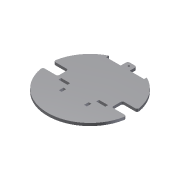
# Autodesk Inventor part: OpenROV_Dev_EChassis_Pivot_Plate
Saved by Autodesk Inventor 2012 (Build 160160000, 160)
## iProperties
Created: 2012-08-08
Part Number: OpenROV_Dev_EChassis_Pivot_Plate
Material: Default
Document SubType Name: Modeling
Designer: user
Density: 1 g/cm^3
Author: user
Autodesk Inventor part; units mm, degrees
ref_plane "YZ Plane" through (0, 0, 0) normal (1, 0, 0) x (0, 1, 0)
ref_plane "XZ Plane" through (0, 0, 0) normal (0, 1, 0) x (-1, 0, 0)
ref_plane "XY Plane" through (0, 0, 0) normal (0, 0, 1) x (1, 0, 0)
sketch "Sketch1" plane through (0, 0, 0) normal (0, 0, 1) x (1, 0, 0)
  line L0 (-26, -6) -> (-16, -6)
  line L1 (-16, -6) -> (-16, -9)
  line L2 (-16, -9) -> (-26, -9)
  line L3 (-26, -9) -> (-26, -6)
  line L4 (16, -6) -> (26, -6)
  line L5 (26, -6) -> (26, -9)
  line L6 (26, -9) -> (16, -9)
  line L7 (16, -9) -> (16, -6)
  line L8 (-15.5, -14) -> (-12.5, -14)
  line L9 (-12.5, -14) -> (-12.5, -19)
  line L10 (-12.5, -19) -> (-15.5, -19)
  line L11 (-15.5, -19) -> (-15.5, -14)
  line L12 (12.5, -14) -> (15.5, -14)
  line L13 (15.5, -14) -> (15.5, -19)
  line L14 (15.5, -19) -> (12.5, -19)
  line L15 (12.5, -19) -> (12.5, -14)
  arc A0 (31.6739, 34.7241) -> (21, 42.0476) centre (0, 0) ccw
  arc A1 (-28.2, 37.6) -> (-31.6739, 34.7241) centre (0, 0) ccw
  line L16 (21, 42.0476) -> (21, 39.0476)
  line L17 (21, 39.0476) -> (5, 39.0476)
  line L18 (-21, 42.0476) -> (-21, 39.0476)
  line L19 (-21, 39.0476) -> (-5, 39.0476)
  line L20 (-5, 39.0476) -> (-5, 44.8999)
  line L21 (5, 39.0476) -> (5, 44.8999)
  arc A2 (3.1333, 46.8954) -> (-3.1333, 46.8954) centre (0, 0) ccw
  circle A3 centre (0, 43.0476) radius 1
  arc A4 (-3.1333, 46.8954) -> (-5, 44.8999) centre (-3, 44.8999) ccw
  arc A5 (5, 44.8999) -> (3.1333, 46.8954) centre (3, 44.8999) ccw
  line L22 (-44.2832, -6) -> (-32, -6)
  line L23 (-30, -4) -> (-30, 4)
  line L24 (-32, 6) -> (-44.2832, 6)
  arc A6 (-21, 42.0476) -> (-46.2513, 8.3556) centre (0, 0) ccw
  line L25 (44.2832, 6) -> (32, 6)
  line L26 (30, 4) -> (30, -4)
  line L27 (32, -6) -> (44.2832, -6)
  arc A7 (-46.2513, -8.3556) -> (46.2513, -8.3556) centre (0, 0) ccw
  arc A8 (46.2513, 8.3556) -> (28.2, 37.6) centre (0, 0) ccw
  arc A9 (44.2832, 6) -> (46.2513, 8.3556) centre (44.2832, 8) ccw
  arc A10 (32, 6) -> (30, 4) centre (32, 4) ccw
  arc A11 (30, -4) -> (32, -6) centre (32, -4) ccw
  arc A12 (46.2513, -8.3556) -> (44.2832, -6) centre (44.2832, -8) ccw
  arc A13 (-46.2513, 8.3556) -> (-44.2832, 6) centre (-44.2832, 8) ccw
  arc A14 (-30, 4) -> (-32, 6) centre (-32, 4) ccw
  arc A15 (-32, -6) -> (-30, -4) centre (-32, -4) ccw
  arc A16 (-44.2832, -6) -> (-46.2513, -8.3556) centre (-44.2832, -8) ccw
  point P0 (-5, 46.7333)
  point P1 (5, 46.7333)
  point P2 (-46.6154, -6)
  point P3 (-46.6154, 6)
  point P4 (46.6154, -6)
  point P5 (46.6154, 6)
  dimension "d3" = 10
  dimension "d4" = 10
  dimension "d5" = 3
  dimension "d6" = 3
  dimension "d7" = 32
  dimension "d8" = 16
  dimension "d12" = 6
  dimension "d13" = 6
  dimension "d14" = 3
  dimension "d15" = 5
  dimension "d16" = 5
  dimension "d17" = 3
  dimension "d18" = 25
  dimension "d19" = 12.5
  dimension "d20" = 5
  dimension "d21" = 5
  dimension "d30" = 3
  dimension "d31" = 3
  dimension "d37" = 47
  dimension "d38" = 10
  dimension "d39" = 16
  dimension "d40" = 16
  dimension "d41" = 2
  dimension "d42" = 4
  dimension "d43" = 5
  dimension "d44" = 5
  dimension "d45" = 2
  dimension "d46" = 30
  dimension "d47" = 30
  dimension "d48" = 2
  constraints: 56 end point, 40 point on circle, 20 tangent, 17 centre point, 12 parallel, 10 perpendicular, 8 equal radius, 6 horizontal, 6 point on line, 2 coincident
  measures "d3" distance between parallel lines of L1 L3
  measures "d4" distance between parallel lines of L5 L7
  measures "d5" distance between parallel lines of L2 L0
  measures "d6" distance between parallel lines of L6 L4
  measures "d7" distance between parallel lines of L7 L1
  measures "d8" distance from line of point (0, 0) L7
  measures "d12" distance from line of point (0, 0) L0
  measures "d13" distance from line of point (0, 0) L4
  measures "d14" distance between parallel lines of L9 L11
  measures "d15" distance between parallel lines of L10 L8
  measures "d16" distance between parallel lines of L14 L12
  measures "d17" distance between parallel lines of L13 L15
  measures "d18" distance between parallel lines of L15 L9
  measures "d19" distance from line of point (0, 0) L9
  measures "d20" distance between parallel lines of L2 L8
  measures "d21" distance between parallel lines of L12 L6
  measures "d30" distance from line of L19 L18.start
  measures "d31" distance from line of L16.start L17
  measures "d37" radius of A2
  measures "d38" distance between parallel lines of L21 L20
  measures "d39" distance between parallel lines of L20 L18
  measures "d40" distance between parallel lines of L16 L21
  measures "d41" diameter of A3
  measures "d42" distance from line of L19 A3.centre
  measures "d43" distance from line of point (0, 0) L20
  measures "d44" distance from line of L20 A3.centre
  measures "d45" radius of A4
  measures "d46" distance from line of point (0, 0) L23
  measures "d47" distance from line of L26 point (0, 0)
  measures "d48" radius of A9
extrude "Extrusion2" add sketch "Sketch1" along normal blind 3
body "Solid2"
